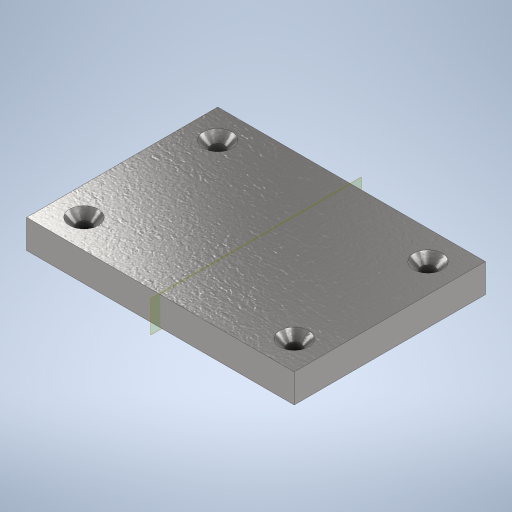
# Autodesk Inventor part: Zylinderkopf
Saved by Autodesk Inventor 2024 (Build 280153000, 153)
## iProperties
Created: 2024-01-15
Part Number: Zylinderkopf
Material: Stahl, galvanisiert
Document SubType Name: Modeling
Designer: ffogue
Density: 7.85 g/cm^3
Appearance: Galvanisiert
Author: ffogue
Autodesk Inventor part; units mm, degrees
ref_plane "XZ Plane" through (0, 0, 0) normal (0, 1, 0) x (-1, 0, 0)
ref_plane "XY Plane" through (0, 0, 0) normal (0, 0, 1) x (1, 0, 0)
sketch "Skizze1" plane through (0, 0, 0) normal (0, 0, 1) x (1, 0, 0)
  line L0 (0, 20) -> (28, 20)
  line L1 (28, 20) -> (28, 0)
  line L2 (28, 0) -> (0, 0)
  line L3 (0, 0) -> (0, 20)
  dimension "d0" = 28
  dimension "d1" = 20
  constraints: 8 end point, 2 parallel, 1 coincident, 1 horizontal, 1 perpendicular
  measures "d0" distance between parallel lines of L1 L3
  measures "d1" distance between parallel lines of L2 L0
extrude "Extrusion1" add sketch "Skizze1" along normal blind 3
sketch "Skizze2" plane through (0, 0, 3) normal (0, 0, 1) x (1, 0, 0)
  line L0 (0, 20) -> (0, 0) projected
  line L1 (0, 10) -> (28.5763, 10) construction
  point P0 (3, 17)
  point P1 (3, 3)
  dimension "d4" = 14
  dimension "d5" = 3
  constraints: 2 end point, 1 horizontal, 1 midpoint, 1 symmetric about line
  measures "d4" distance of point (3, 3) point (3, 17)
  measures "d5" distance from line of point (3, 17) L0
hole "Bohrung1" at (3, 17, 3) at (3, 3, 3) direction (0, 0, -1) diameter 1.4 end through all countersink diameter 3 countersink angle 90
ref_plane "Arbeitsebene1" through (14, 0, 0) normal (1, 0, 0) x (0, 1, 0)
mirror "Spiegeln1" about plane through (14, 0, 0) normal (1, 0, 0) of "Bohrung1"
ref_plane "Arbeitsebene2" through (14, 0, 0) normal (1, 0, 0) x (0, 1, 0)
